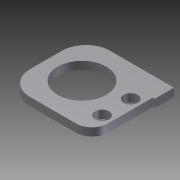
# Autodesk Inventor part: suport sensor proximitat
Saved by Autodesk Inventor 2012 SP1 (Build 160190100, 190)
## iProperties
Created: 2015-03-26
Part Number: suport sensor proximitat
Material: Default
Document SubType Name: Modeling
Designer: Laser router cnc
Density: 1 g/cm^3
Author: Laser router cnc
Autodesk Inventor part; units mm, degrees
ref_plane "YZ Plane" through (0, 0, 0) normal (1, 0, 0) x (0, 1, 0)
ref_plane "XZ Plane" through (0, 0, 0) normal (0, 1, 0) x (-1, 0, 0)
ref_plane "XY Plane" through (0, 0, 0) normal (0, 0, 1) x (1, 0, 0)
sketch "Boceto1" plane through (0, 0, 0) normal (0, 0, 1) x (1, 0, 0)
  line L0 (-10.7186, 2.8144) -> (9.2814, 2.8144)
  line L1 (9.2814, 2.8144) -> (9.2814, -17.1856)
  line L2 (9.2814, -17.1856) -> (-10.7186, -17.1856)
  line L3 (-10.7186, -17.1856) -> (-10.7186, 2.8144)
  point P0 (0, 0)
  dimension "d0" = 20
  dimension "d1" = 20
  constraints: 8 end point, 2 parallel, 1 horizontal, 1 perpendicular
  measures "d0" distance of L1.end L2.end
  measures "d1" distance of L0.end L1.end
extrude "Extrusión1" add sketch "Boceto1" along normal blind 2
sketch "Boceto2" plane through (0, 0, 2) normal (0, 0, 1) x (1, 0, 0)
  line L0 (-10.7186, 2.8144) -> (9.2814, 2.8144) projected
  line L1 (-10.7186, -17.1856) -> (-10.7186, 2.8144) projected
  circle A0 centre (-3.7186, -7.1856) radius 6.1
  point P0 (0, 0)
  dimension "d4" = 12.2
  dimension "d5" = 7
  dimension "d6" = 10
  constraints: 1 centre point
  measures "d4" diameter of A0
  measures "d5" distance from line of L1 A0.centre
  measures "d6" distance from line of L0 A0.centre
extrude "Extrusión2" cut sketch "Boceto2" against normal blind 5
move faces "Desplazar cara1" translate (-2, 0, 0) faces at (-10.7186, -10.519, 0.6667)
sketch "Boceto3" plane through (0, 0, 2) normal (0, 0, 1) x (1, 0, 0)
  line L0 (9.2814, 2.8144) -> (9.2814, -17.1856) projected
  line L1 (12.9791, -1.9852) -> (8.7814, -1.9852)
  line L2 (8.7814, -1.9852) -> (8.7814, -18.2161)
  line L3 (8.7814, -18.2161) -> (12.9791, -18.2161)
  line L4 (12.9791, -18.2161) -> (12.9791, -1.9852)
  point P0 (0, 0)
  dimension "d9" = 0.5
  constraints: 8 end point, 2 parallel, 1 horizontal, 1 perpendicular
  measures "d9" distance between parallel lines of L0 L2
extrude "Extrusión3" cut sketch "Boceto3" against normal blind 5
fillet "Empalme1" radius 6 2 edges at (-12.7186, 2.8144, 1) (-12.7186, -17.1856, 1)
fillet "Empalme2" radius 4 1 edges at (8.7814, -17.1856, 1)
sketch "Boceto4" plane through (0, 0, 2) normal (0, 0, 1) x (1, 0, 0)
  line L0 (8.7814, -13.1856) -> (8.7814, -1.9852) projected
  circle A0 centre (6.2814, -5.0231) radius 1.75
  circle A1 centre (6.2814, -12.1666) radius 1.75
  point P0 (0, 0)
  dimension "d14" = 3.5
  dimension "d15" = 3.5
  dimension "d16" = 2.5
  dimension "d17" = 2.5
  constraints: 2 centre point
  measures "d14" diameter of A0
  measures "d15" diameter of A1
  measures "d16" distance from line of L0 A0.centre
  measures "d17" distance from line of L0 A1.centre
extrude "Extrusión4" cut sketch "Boceto4" against normal blind 5
